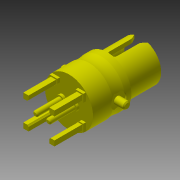
# Autodesk Inventor part: CJT-T-P-HH-ST-TH1
Saved by Autodesk Inventor 2014 SP2 (Build 180246200, 246)
## iProperties
Created: 2018-08-02
Part Number: CJT-T-P-HH-ST-TH1
Material: Generic
Catalog Web Link: www.cadenas.de
Description: CJT-TH Series-Circular RF Twinax Jack, Through-hole
Vendor: SAMTEC
Document SubType Name: Modeling
Designer: psadmin
Manufacturer: SAMTEC
Mass: 0.0833247 g
Surface Area: 2.03707 cm^2
Volume: 0.0833247 cm^3
Density: 1 g/cm^3
Appearance: PSOLRGB-255-255-0
Category: PARTsolutions
Company: SAMTEC
Title: CJT-T-P-HH-ST-TH1
Author: Cadenas PARTsolutions
Comments: Circular RF Twinax Jack, Through-hole
PSOL_IDENT_0: {$CADENAS_DATA\23d-libs\samtec\modelling\cjt\cjt-th.prj},190 {VTYP=3D},{NB=CJT-T-P-HH-ST-TH1},{LINA=
PSOL_IDENT_1: CJT-T-P-HH-ST-TH1},{NN=CJT-TH Series},{DATE=26.10.2016 12:02:31},{GEOMDATE=19.09.2016 12:10:38},{VER
PSOL_IDENT_2: SION=},{LINEID=10},{WBVAR=PLOPT,ORI},{WBNUMERIC=}  {NB=CJT-T-P-HH-ST-TH1},{LINA=CJT-T-P-HH-ST-TH1},{
PSOL_IDENT_3: KT=DUMMY},{PN=CJT-T-P-HH-ST-TH1},{SERIES=CJT-TH},{GEN=-T: Terminal},{TYPE=-P: PCB},{PLOPT=HH},{PLOPT
PSOL_IDENT_4: ALG= 'HH','-HH: Heavy Gold / Heavy Gold 30 µ\" Au / 50 µ\" Ni Min on Pin 30 µ\" Au / 50 µ\" Ni Min o
PSOL_IDENT_5: n Outer Contact','GF','Non-standard option - Please contact SAMTEC: -GF: Gold / Flash Gold 10 µ\" Au
PSOL_IDENT_6: / 50 µ\" Ni Min on Pin 3 µ\" Au / 50 µ\" Ni Min on Outer Contact' },{ORI=ST},{TERM=-TH1: Through Ho
PSOL_IDENT_7: le}
NN: CJT-TH Series
NT: Circular RF Twinax Jack, Through-hole
NB: CJT-T-P-HH-ST-TH1
NBSYN: $PN.
LINA: CJT-T-P-HH-ST-TH1
PN: CJT-T-P-HH-ST-TH1
SERIES: CJT-TH
GEN: -T: Terminal
TYPE: -P: PCB
PLOPT: -HH: Heavy Gold / Heavy Gold 30 µ" Au / 50 µ" Ni Min on Pin 30 µ" Au / 50 µ" Ni Min on Outer Contact
ORI: -ST: Straight
TERM: -TH1: Through Hole
SUPPLIER: SAMTEC
ARTICLENO: CJT-T-P-HH-ST-TH1
BOMINFO: CJT-T-P-HH-ST-TH1
CREATOR: CADENAS GmbH
Autodesk Inventor part; units mm, degrees
ref_plane "YZ Plane" through (0, 0, 0) normal (1, 0, 0) x (0, 1, 0)
ref_plane "XZ Plane" through (0, 0, 0) normal (0, 1, 0) x (-1, 0, 0)
ref_plane "XY Plane" through (0, 0, 0) normal (0, 0, 1) x (1, 0, 0)
sketch "Sketch0" plane through (0, 0, 0) normal (1, 0, 0) x (0, 0, -1)
  line L0 (0, -2.95) -> (0, 3.76)
  line L1 (0, 3.76) -> (1.575, 3.76)
  line L2 (1.575, 3.76) -> (1.575, 6.6347)
  line L3 (1.575, 6.6347) -> (1.65, 7.06)
  line L4 (1.65, 7.06) -> (1.97, 7.06)
  line L5 (1.97, 7.06) -> (1.97, 3.76)
  line L6 (1.97, 3.76) -> (2.35, 3.76)
  line L7 (2.35, 3.76) -> (2.35, 3.115)
  arc A0 (2.35, 3.115) -> (2.35, 1.965) centre (4.6766, 2.54) ccw
  line L8 (2.35, 1.965) -> (2.35, -2.95)
  line L9 (2.35, -2.95) -> (0, -2.95)
  line L10 (0, -2.95) -> (0, 3.76)
  constraints: 22 end point, 2 point on circle, 1 centre point
revolve "Revolution1" add sketch "Sketch0" angle 360 about axis through (0, -2.95, 0) along (0, -1, 0)
sketch "Sketch2" plane through (0, -0.254, 0) normal (0, -1, 0) x (1, 0, 0)
  line L0 (-2.8207, -2.5724) -> (2.7363, -2.5724)
  line L1 (2.7363, -2.5724) -> (2.7363, 2.5607)
  line L2 (2.7363, 2.5607) -> (-2.8207, 2.5607)
  line L3 (-2.8207, 2.5607) -> (-2.8207, -2.5724)
  line L4 (1.015, 1.525) -> (1.015, 1.1382)
  arc A0 (1.1382, 1.015) -> (1.015, 1.1382) centre (0, 0) ccw
  line L5 (1.1382, 1.015) -> (1.525, 1.015)
  line L6 (1.525, 1.015) -> (1.525, 1.525)
  line L7 (1.525, 1.525) -> (1.015, 1.525)
  line L8 (1.015, -1.525) -> (1.525, -1.525)
  line L9 (1.525, -1.525) -> (1.525, -1.015)
  line L10 (1.525, -1.015) -> (1.1382, -1.015)
  arc A1 (1.015, -1.1382) -> (1.1382, -1.015) centre (0, 0) ccw
  line L11 (1.015, -1.1382) -> (1.015, -1.525)
  line L12 (-1.525, 1.015) -> (-1.1382, 1.015)
  arc A2 (-1.015, 1.1382) -> (-1.1382, 1.015) centre (0, 0) ccw
  line L13 (-1.015, 1.1382) -> (-1.015, 1.525)
  line L14 (-1.015, 1.525) -> (-1.525, 1.525)
  line L15 (-1.525, 1.525) -> (-1.525, 1.015)
  line L16 (-1.525, -1.525) -> (-1.015, -1.525)
  line L17 (-1.015, -1.525) -> (-1.015, -1.1382)
  arc A3 (-1.1382, -1.015) -> (-1.015, -1.1382) centre (0, 0) ccw
  line L18 (-1.1382, -1.015) -> (-1.525, -1.015)
  line L19 (-1.525, -1.015) -> (-1.525, -1.525)
  constraints: 40 end point, 8 point on circle, 4 centre point
sketch "Sketch1" plane through (0, 0, 0) normal (0, 0, 1) x (1, 0, 0)
  line L0 (-3.2466, 11.5152) -> (-0.4483, 6.6683)
  arc A0 (-0.38, 6.4133) -> (-0.4483, 6.6683) centre (-0.89, 6.4133) ccw
  line L1 (-0.38, 6.4133) -> (-0.38, 4.34)
  arc A1 (-0.38, 4.34) -> (0.38, 4.34) centre (0, 4.34) ccw
  line L2 (0.38, 4.34) -> (0.38, 6.4133)
  arc A2 (0.4483, 6.6683) -> (0.38, 6.4133) centre (0.89, 6.4133) ccw
  line L3 (0.4483, 6.6683) -> (3.2466, 11.5152)
  line L4 (3.2466, 11.5152) -> (-3.2466, 11.5152)
  constraints: 10 end point, 6 point on circle, 3 centre point
extrude "Extrusion1" cut sketch "Sketch1" along normal blind 2
sketch "Sketch3" plane through (0, 0, 0) normal (0, -1, 0) x (1, 0, 0)
  line L0 (-3.2744, -3.0008) -> (3.3, -3.0008)
  line L1 (3.3, -3.0008) -> (3.3, 2.8478)
  line L2 (3.3, 2.8478) -> (-3.2744, 2.8478)
  line L3 (-3.2744, 2.8478) -> (-3.2744, -3.0008)
  line L4 (0.89, 1.65) -> (0.89, 1.2384)
  arc A0 (1.2384, 0.89) -> (0.89, 1.2384) centre (0, 0) ccw
  line L5 (1.2384, 0.89) -> (1.65, 0.89)
  line L6 (1.65, 0.89) -> (1.65, 1.65)
  line L7 (1.65, 1.65) -> (0.89, 1.65)
  line L8 (0.89, -1.65) -> (1.65, -1.65)
  line L9 (1.65, -1.65) -> (1.65, -0.89)
  line L10 (1.65, -0.89) -> (1.2384, -0.89)
  arc A1 (0.89, -1.2384) -> (1.2384, -0.89) centre (0, 0) ccw
  line L11 (0.89, -1.2384) -> (0.89, -1.65)
  line L12 (-1.65, 0.89) -> (-1.2384, 0.89)
  arc A2 (-0.89, 1.2384) -> (-1.2384, 0.89) centre (0, 0) ccw
  line L13 (-0.89, 1.2384) -> (-0.89, 1.65)
  line L14 (-0.89, 1.65) -> (-1.65, 1.65)
  line L15 (-1.65, 1.65) -> (-1.65, 0.89)
  line L16 (-1.65, -1.65) -> (-0.89, -1.65)
  line L17 (-0.89, -1.65) -> (-0.89, -1.2384)
  arc A3 (-1.2384, -0.89) -> (-0.89, -1.2384) centre (0, 0) ccw
  line L18 (-1.2384, -0.89) -> (-1.65, -0.89)
  line L19 (-1.65, -0.89) -> (-1.65, -1.65)
  constraints: 40 end point, 8 point on circle, 4 centre point
extrude "Extrusion2" cut sketch "Sketch2" along normal blind 2.696
sketch "Sketch4" plane through (-2.2, 0, 0) normal (-1, 0, 0) x (0, 0, 1)
  circle A0 centre (0, 2.54) radius 0.75
  constraints: 1 centre point
extrude "Extrusion3" cut sketch "Sketch3" along normal blind 2.95
sketch "Sketch5" plane through (2.2, 0, 0) normal (1, 0, 0) x (0, 0, -1)
  circle A0 centre (0, 2.54) radius 0.75
  constraints: 1 centre point
extrude "Extrusion4" cut sketch "Sketch4" along normal blind 0.5
sketch "Sketch6" plane through (0, 0, 0) normal (0, 0, 1) x (1, 0, 0)
  line L0 (-0.6355, 6.35) -> (-0.6355, -2.7)
  line L1 (-0.6355, -2.7) -> (-0.7874, -2.7)
  line L2 (-0.7874, -2.7) -> (-0.889, -2.5984)
  line L3 (-0.889, -2.5984) -> (-0.889, -0.25)
  line L4 (-0.889, -0.25) -> (-1.015, -0.25)
  line L5 (-1.015, -0.25) -> (-1.015, 3.76)
  line L6 (-1.015, 3.76) -> (-0.8882, 3.76)
  line L7 (-0.8882, 3.76) -> (-0.8382, 3.81)
  line L8 (-0.8382, 3.81) -> (-0.8255, 3.81)
  line L9 (-0.8255, 3.81) -> (-0.8255, 6.16)
  arc A0 (-0.6355, 6.35) -> (-0.8255, 6.16) centre (-0.6355, 6.16) ccw
  line L10 (-0.6355, 6.35) -> (-0.6355, -2.7)
  constraints: 22 end point, 2 point on circle, 1 centre point
extrude "Extrusion5" cut sketch "Sketch5" along normal blind 0.5
sketch "Sketch7" plane through (0, 0, 0) normal (0, 0, 1) x (1, 0, 0)
  line L0 (0.6345, -2.7) -> (0.6345, 6.35)
  arc A0 (0.8255, 6.16) -> (0.6345, 6.35) centre (0.6355, 6.16) ccw
  line L1 (0.8255, 6.16) -> (0.8255, 3.81)
  line L2 (0.8255, 3.81) -> (0.8382, 3.81)
  line L3 (0.8382, 3.81) -> (0.8882, 3.76)
  line L4 (0.8882, 3.76) -> (1.015, 3.76)
  line L5 (1.015, 3.76) -> (1.015, -0.25)
  line L6 (1.015, -0.25) -> (0.889, -0.25)
  line L7 (0.889, -0.25) -> (0.889, -2.5984)
  line L8 (0.889, -2.5984) -> (0.7874, -2.7)
  line L9 (0.7874, -2.7) -> (0.6345, -2.7)
  line L10 (0.6345, -2.7) -> (0.6345, 6.35)
  constraints: 22 end point, 2 point on circle, 1 centre point
revolve "Revolution2" add sketch "Sketch6" angle 360 about axis through (-0.6355, 6.35, 0) along (0, 1, 0)
sketch "Sketch8" plane through (0, 0, 0) normal (0, 0, 1) x (1, 0, 0)
  line L0 (3.175, 2.54) -> (-3.175, 2.54)
  line L1 (-3.175, 2.54) -> (-3.175, 2.79)
  line L2 (-3.175, 2.79) -> (-3.075, 2.89)
  line L3 (-3.075, 2.89) -> (3.075, 2.89)
  line L4 (3.075, 2.89) -> (3.175, 2.79)
  line L5 (3.175, 2.79) -> (3.175, 2.54)
  line L6 (3.175, 2.54) -> (-3.175, 2.54)
  constraints: 14 end point
revolve "Revolution3" add sketch "Sketch7" angle 360 about axis through (0.6345, -2.7, 0) along (0, -1, 0)
revolve "Revolution4" add sketch "Sketch8" angle 360 about axis through (3.175, 2.54, 0) along (1, 0, 0)
body "Solid1"
